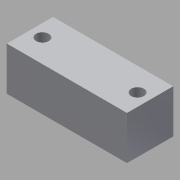
# Autodesk Inventor part: 2.5 CIM mount
Saved by Autodesk Inventor 2013 (Build 170138000, 138)
## iProperties
Created: 2013-01-18
Part Number: 2.5 CIM mount
Material: ABS Plastic
Document SubType Name: Modeling
Designer: Naphat
Density: 1 g/cm^3
Author: Naphat
Autodesk Inventor part; units mm, degrees
ref_plane "YZ Plane" through (0, 0, 0) normal (1, 0, 0) x (0, 1, 0)
ref_plane "XZ Plane" through (0, 0, 0) normal (0, 1, 0) x (-1, 0, 0)
ref_plane "XY Plane" through (0, 0, 0) normal (0, 0, 1) x (1, 0, 0)
sketch "Sketch20" plane through (0, 0, 0) normal (0, 1, 0) x (-1, 0, 0)
  line L0 (56.8325, -21.844) -> (-56.8325, -21.844)
  line L1 (-56.8325, -21.844) -> (-56.8325, 21.844)
  line L2 (-56.8325, 21.844) -> (56.8325, 21.844)
  line L3 (56.8325, 21.844) -> (56.8325, -21.844)
  circle A0 centre (45, 0) radius 6
  circle A1 centre (-45, 0) radius 6
  point P0 (0, 0)
  dimension "d92" = 113.665
  dimension "d93" = 43.688
  dimension "d94" = 56.8325
  dimension "d95" = 21.844
  dimension "d97" = 45
  dimension "d98" = 90
  dimension "d99" = 12
  dimension "d100" = 12
  constraints: 8 end point, 2 centre point, 2 horizontal alignment, 2 parallel, 1 horizontal, 1 perpendicular
  measures "d92" distance between parallel lines of L3 L1
  measures "d93" distance between parallel lines of L0 L2
  measures "d94" distance from line of point (0, 0) L3
  measures "d95" distance from line of point (0, 0) L2
  measures "d97" distance of A1.centre point (0, 0)
  measures "d98" distance of A1.centre A0.centre
  measures "d99" diameter of A0
  measures "d100" diameter of A1
extrude "Extrusion17" add sketch "Sketch20" along normal blind 41.0718
equation "\"d94\" = 0.5 * d92"
equation "\"d95\" = 0.5 * d93"
equation "\"d97\" = 0.5 * d98"
equation "\"d100\" = d99"
body "Solid3"
